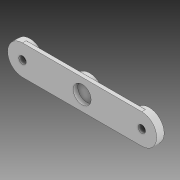
# Autodesk Inventor part: Cablecar_pulleybracket
Saved by Autodesk Inventor 2020 (Build 240168000, 168)
## iProperties
Created: 2021-02-03
Part Number: Cablecar_pulleybracket
Material: Generic
Document SubType Name: Modeling
Designer: DDeGo
Density: 1 g/cm^3
Appearance: Default
Author: DDeGo
Autodesk Inventor part; units mm, degrees
ref_plane "YZ Plane" through (0, 0, 0) normal (1, 0, 0) x (0, 1, 0)
ref_plane "XZ Plane" through (0, 0, 0) normal (0, 1, 0) x (-1, 0, 0)
ref_plane "XY Plane" through (0, 0, 0) normal (0, 0, 1) x (1, 0, 0)
sketch "Sketch1" plane through (0, 0, 0) normal (0, 0, 1) x (1, 0, 0)
  line L0 (40, 0) -> (-40, 0) construction
  line L1 (40, 10) -> (-40, 10)
  line L2 (-40, -10) -> (40, -10)
  arc A0 (40, -10) -> (40, 10) centre (40, 0) ccw
  arc A1 (-40, 10) -> (-40, -10) centre (-40, 0) ccw
  circle A2 centre (-40, 0) radius 2.5 construction
  circle A3 centre (40, 0) radius 2.5 construction
  point P0 (0, 0)
  dimension "d0" = 5
  dimension "d1" = 20
  dimension "d2" = 80
  constraints: 8 end point, 4 centre point, 4 point on circle, 4 tangent, 2 coincident, 1 equal radius, 1 horizontal, 1 midpoint, 1 parallel
  measures "d0" diameter of A2
  measures "d1" distance between parallel lines of L2 L1
  measures "d2" distance of L0.start L0.end
extrude "Extrusion1" add sketch "Sketch1" along normal blind 2.5
sketch "Sketch2" plane through (0, 0, 0) normal (0, 1, 0) x (-1, 0, 0)
  line L0 (0, 0) -> (0, -8)
  line L1 (0, -8) -> (-2.4, -8)
  line L2 (40, 0) -> (-40, 0) projected
  line L3 (0, 0) -> (-3.4, 0)
  line L4 (-3.4, 0) -> (-3.4, -3.5)
  line L5 (-3.4, -3.5) -> (-2.4, -3.5)
  line L6 (-2.4, -3.5) -> (-2.4, -8)
  dimension "d5" = 2.4
  dimension "d6" = 4.5
  dimension "d7" = 1
  dimension "d8" = 3.5
  constraints: 12 end point, 3 perpendicular, 2 vertical, 1 point on line
  measures "d5" distance between parallel lines of L0 L6
  measures "d6" distance between parallel lines of L1 L5
  measures "d7" distance of L4.end L5.end
  measures "d8" distance between parallel lines of L2 L5
revolve "Revolution1" add sketch "Sketch2" angle 360 about axis through (0, 0, 0) along (0, 0, -1)
sketch "Sketch3" plane through (0, 0, 0) normal (0, 0, -1) x (-1, 0, 0)
  circle A0 centre (0, 0) radius 3.4 projected
  arc A1 (40, -10) -> (40, 10) centre (40, 0) ccw projected
  line L0 (-40, 10) -> (40, 10) projected
  arc A2 (-40, 10) -> (-40, -10) centre (-40, 0) ccw projected
  line L1 (40, -10) -> (-40, -10) projected
  circle A3 centre (-40, 0) radius 10
  circle A4 centre (0, 0) radius 3.4 projected
  circle A5 centre (0, 0) radius 10
  circle A6 centre (40, 0) radius 10
  point P0 (-40, -10)
  dimension "d10" = 20
  constraints: 3 centre point, 3 coincident, 2 equal radius
  measures "d10" diameter of A5
extrude "Extrusion2" add sketch "Sketch3" along normal blind 2.5 contours A0 | A6 A1 | A5 | A2 A3
sketch "Sketch4" plane through (0, 0, 2.5) normal (0, 0, 1) x (1, 0, 0)
  arc A0 (-40, 10) -> (-40, -10) centre (-40, 0) ccw projected
  line L0 (-40, -10) -> (40, -10) projected
  arc A1 (40, -10) -> (40, 10) centre (40, 0) ccw projected
  line L1 (40, 10) -> (-40, 10) projected
  circle A2 centre (40, 0) radius 2.5
  circle A3 centre (0, 0) radius 6
  circle A4 centre (-40, 0) radius 2.5
  dimension "d13" = 12
  dimension "d14" = 5
  dimension "d15" = 5
  constraints: 3 centre point, 3 coincident
  measures "d13" diameter of A3
  measures "d14" diameter of A2
  measures "d15" diameter of A4
extrude "Extrusion3" cut sketch "Sketch4" against normal blind 3 contours A2 | A3 | A4
body "Solid1"
